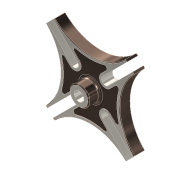
# Autodesk Inventor part: Malta Cross
Saved by Autodesk Inventor 2022.2 (Build 262287010, 287A)
## iProperties
Created: 2022-12-20
Part Number: Malta Cross
Material: Steel
Document SubType Name: Modeling
Designer: User
Density: 7.85 g/cm^3
Appearance: Gunmetal - Antique Polished
Mass: 222.814 g
Surface Area: 117.925 cm^2
Volume: 28.384 cm^3
Author: User
Autodesk Inventor part; units mm, degrees
ref_plane "YZ Plane" through (0, 0, 0) normal (1, 0, 0) x (0, 1, 0)
ref_plane "XZ Plane" through (0, 0, 0) normal (0, 1, 0) x (-1, 0, 0)
ref_plane "XY Plane" through (0, 0, 0) normal (0, 0, 1) x (1, 0, 0)
sketch "Sketch1" plane through (0, 0, 0) normal (0, 0, 1) x (1, 0, 0)
  circle A0 centre (0, 0) radius 51.6188
  dimension "d0" = 103.2376
  constraints: 1 centre point, 1 coincident
  measures "d0" diameter of A0
extrude "Extrusion1" add sketch "Sketch1" along normal mid plane 10
sketch "Sketch2" plane through (0, 0, 5) normal (0, 0, 1) x (1, 0, 0)
  circle A0 centre (0, 0) radius 51.6188 projected
  arc A1 (-32.3092, 40.2568) -> (32.3092, 40.2568) centre (0, 73) ccw
  line L0 (0, 0) -> (36.5, 36.5) construction
  line L1 (0, -76.5426) -> (0, 97.9238) construction
  arc A2 (11.5258, 16.7584) -> (16.7584, 11.5258) centre (14.1421, 14.1421) ccw
  line L2 (11.5258, 16.7584) -> (33.7898, 39.0224)
  line L3 (16.7584, 11.5258) -> (39.0224, 33.7898)
  dimension "d3" = 46
  dimension "d4" = 73
  dimension "d5" = 20
  dimension "d6" = 45
  dimension "d7" = 3.7
  constraints: 9 point on circle, 6 end point, 2 centre point, 2 parallel, 2 tangent, 1 coincident, 1 point on line, 1 vertical alignment
  measures "d3" radius of A1
  measures "d4" distance of L0.start A1.centre
  measures "d5" distance of L0.start point (14.142, 14.142)
  measures "d6" angle of L0 L1
  measures "d7" radius of A2
extrude "Extrusion2" cut sketch "Sketch2" against normal through all contours L3 A2 L2 A0 | A0 A1
pattern_circular "Circular Pattern1" count 4 over 360 about axis through (0, 0, 0) along (0, 0, 1) of "Extrusion2"
chamfer "Chamfer1" distance 0.5 angle 45 8 edges at (0, 27, -5) (0, 27, 5) (27, 0, 5) (27, 0, -5) (-27, 0, 5) (0, -27, 5) (-27, 0, -5) (0, -27, -5)
sketch "Sketch3" plane through (0, 0, 5) normal (0, 0, 1) x (1, 0, 0)
  arc A0 (32.7, -39.9401) -> (-32.7, -39.9401) centre (0, -73) ccw projected
  line L0 (33.7898, -39.0224) -> (11.5258, -16.7584) projected
  arc A1 (16.7584, -11.5258) -> (11.5258, -16.7584) centre (14.1421, -14.1421) ccw projected
  line L1 (16.7584, -11.5258) -> (39.0224, -33.7898) projected
  arc A2 (39.9401, 32.7) -> (39.9401, -32.7) centre (73, 0) ccw projected
  line L2 (39.0224, 33.7898) -> (16.7584, 11.5258) projected
  arc A3 (11.5258, 16.7584) -> (16.7584, 11.5258) centre (14.1421, 14.1421) ccw projected
  line L3 (11.5258, 16.7584) -> (33.7898, 39.0224) projected
  arc A4 (-32.7, 39.9401) -> (32.7, 39.9401) centre (0, 73) ccw projected
  line L4 (-33.7898, 39.0224) -> (-11.5258, 16.7584) projected
  arc A5 (-16.7584, 11.5258) -> (-11.5258, 16.7584) centre (-14.1421, 14.1421) ccw projected
  line L5 (-16.7584, 11.5258) -> (-39.0224, 33.7898) projected
  arc A6 (-39.9401, -32.7) -> (-39.9401, 32.7) centre (-73, 0) ccw projected
  line L6 (-39.0224, -33.7898) -> (-16.7584, -11.5258) projected
  arc A7 (-11.5258, -16.7584) -> (-16.7584, -11.5258) centre (-14.1421, -14.1421) ccw projected
  line L7 (-11.5258, -16.7584) -> (-33.7898, -39.0224) projected
  line L8 (14.843, 22.904) -> (10.1116, 18.1726)
  arc A8 (10.1116, 18.1726) -> (18.1726, 10.1116) centre (14.1421, 14.1421) ccw
  line L9 (18.1726, 10.1116) -> (22.904, 14.843)
  arc A9 (26.2462, 12.8969) -> (26.2462, -12.8969) centre (73, 0) ccw
  line L10 (22.904, -14.843) -> (18.1726, -10.1116)
  arc A10 (18.1726, -10.1116) -> (10.1116, -18.1726) centre (14.1421, -14.1421) ccw
  line L11 (10.1116, -18.1726) -> (14.843, -22.904)
  arc A11 (12.8969, -26.2462) -> (-12.8969, -26.2462) centre (0, -73) ccw
  line L12 (-14.843, -22.904) -> (-10.1116, -18.1726)
  arc A12 (-10.1116, -18.1726) -> (-18.1726, -10.1116) centre (-14.1421, -14.1421) ccw
  line L13 (-18.1726, -10.1116) -> (-22.904, -14.843)
  arc A13 (-26.2462, -12.8969) -> (-26.2462, 12.8969) centre (-73, 0) ccw
  line L14 (-22.904, 14.843) -> (-18.1726, 10.1116)
  arc A14 (-18.1726, 10.1116) -> (-10.1116, 18.1726) centre (-14.1421, 14.1421) ccw
  line L15 (-10.1116, 18.1726) -> (-14.843, 22.904)
  arc A15 (-12.8969, 26.2462) -> (12.8969, 26.2462) centre (0, 73) ccw
  arc A16 (-12.8969, 26.2462) -> (-14.843, 22.904) centre (-13.4287, 24.3182) ccw
  arc A17 (14.843, 22.904) -> (12.8969, 26.2462) centre (13.4287, 24.3182) ccw
  arc A18 (26.2462, 12.8969) -> (22.904, 14.843) centre (24.3182, 13.4287) ccw
  arc A19 (22.904, -14.843) -> (26.2462, -12.8969) centre (24.3182, -13.4287) ccw
  arc A20 (12.8969, -26.2462) -> (14.843, -22.904) centre (13.4287, -24.3182) ccw
  arc A21 (-14.843, -22.904) -> (-12.8969, -26.2462) centre (-13.4287, -24.3182) ccw
  arc A22 (-26.2462, -12.8969) -> (-22.904, -14.843) centre (-24.3182, -13.4287) ccw
  arc A23 (-22.904, 14.843) -> (-26.2462, 12.8969) centre (-24.3182, 13.4287) ccw
  point P0 (21.4306, 29.4916)
  point P1 (29.4916, 21.4306)
  point P2 (29.4916, -21.4306)
  point P3 (21.4306, -29.4916)
  point P4 (-21.4306, -29.4916)
  point P5 (-29.4916, -21.4306)
  point P6 (-29.4916, 21.4306)
  point P7 (-21.4306, 29.4916)
  dimension "d16" = 2
  dimension "d17" = 2
  constraints: 40 point on circle, 16 centre point, 16 end point, 16 tangent, 8 point on line, 7 equal radius, 15 other
  measures "d16" radial gap between concentric circles of A4 A15
  measures "d17" radius of A16
extrude "Extrusion3" cut sketch "Sketch3" against normal blind 0.5
mirror "Mirror1" about plane through (0, 0, 0) normal (0, 0, 1) of "Extrusion3"
sketch "Sketch4" plane through (0, 0, 4.5) normal (0, 0, 1) x (1, 0, 0)
  circle A0 centre (0, 0) radius 9
  dimension "d20" = 18
  constraints: 1 centre point, 1 coincident
  measures "d20" diameter of A0
extrude "Extrusion4" add sketch "Sketch4" along normal blind 10.5
sketch "Sketch5" plane through (0, 0, 15) normal (0, 0, 1) x (1, 0, 0)
  circle A0 centre (0, 0) radius 9 projected
  constraints: 1 coincident
hole "Hole1" at (0, 0, 15) direction (0, 0, -1) diameter 9 end through all
fillet "Fillet1" radius 2 1 edges at (-9, 0, 4.5)
chamfer "Chamfer2" distance 1 angle 45 1 edges at (-9, 0, 15)
body "Solid1"
